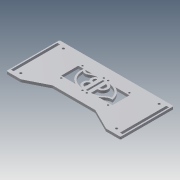
# Autodesk Inventor part: FrontPanel
Saved by Autodesk Inventor 2014 (Build 180170000, 170)
## iProperties
Created: 2015-01-19
Part Number: FrontPanel
Material: Generic
Document SubType Name: Modeling
Designer: Peele
Density: 1 g/cm^3
Appearance: White
Author: Peele
Autodesk Inventor part; units mm, degrees
ref_plane "YZ Plane" through (0, 0, 0) normal (1, 0, 0) x (0, 1, 0)
ref_plane "XZ Plane" through (0, 0, 0) normal (0, 1, 0) x (-1, 0, 0)
ref_plane "XY Plane" through (0, 0, 0) normal (0, 0, 1) x (1, 0, 0)
sketch "Sketch1" plane through (0, 0, 0) normal (0, 0, 1) x (1, 0, 0)
  line L0 (0, 0) -> (0, 125)
  line L1 (0, 125) -> (268, 125)
  line L2 (268, 125) -> (268, 0)
  line L3 (268, 0) -> (0, 0)
  point P0 (134, 125)
  dimension "d1" = 125
  dimension "d2" = 268
  constraints: 8 end point, 2 horizontal, 2 vertical, 1 midpoint
  measures "d1" distance of L1.end L2.end
  measures "d2" distance of L2.end L0.start
extrude "Extrusion1" add sketch "Sketch1" along normal blind 6
sketch "Sketch2" plane through (0, 0, 6) normal (0, 0, 1) x (1, 0, 0)
  line L0 (0, 0) -> (268, 0) projected
  line L1 (268, 0) -> (268, 125) projected
  line L2 (34, 0) -> (84, 25)
  line L3 (84, 25) -> (184, 25)
  line L4 (184, 25) -> (234, 0)
  line L5 (234, 0) -> (34, 0)
  line L6 (0, 125) -> (0, 0) projected
  dimension "d6" = 25
  dimension "d7" = 34
  dimension "d9" = 50
  dimension "d47" = 34
  constraints: 8 end point, 2 point on line, 1 collinear, 1 equal length, 1 parallel
  measures "d6" distance between parallel lines of L0 L3
  measures "d7" distance from line of L4.end L1
  measures "d9" horizontal distance of L2.end L2.start
  measures "d47" distance from line of L6 L2.start
extrude "Extrusion2" cut sketch "Sketch2" against normal through all
sketch "Sketch7" plane through (0, 0, 6) normal (0, 0, 1) x (1, 0, 0)
  line L0 (268, 0) -> (268, 125) projected
  line L1 (268, 125) -> (0, 125) projected
  line L2 (0, 125) -> (0, 0) projected
  line L3 (0, 0) -> (34, 0) projected
  circle A0 centre (246.5, 12.5) radius 2.7
  circle A1 centre (246.5, 112.5) radius 2.7
  circle A2 centre (21.5, 12.5) radius 2.7
  circle A3 centre (21.5, 112.5) radius 2.7
  line L4 (2.875, 8.1) -> (9.125, 8.1)
  line L5 (9.125, 8.1) -> (9.125, 117)
  line L6 (9.125, 117) -> (2.875, 117)
  line L7 (2.875, 117) -> (2.875, 8.1)
  line L8 (2.875, 8.1) -> (9.125, 117) construction
  line L9 (9.125, 8.1) -> (2.875, 117) construction
  line L10 (258.875, 8.1) -> (265.125, 8.1)
  line L11 (265.125, 8.1) -> (265.125, 117)
  line L12 (265.125, 117) -> (258.875, 117)
  line L13 (258.875, 117) -> (258.875, 8.1)
  line L14 (258.875, 8.1) -> (265.125, 117) construction
  line L15 (265.125, 8.1) -> (258.875, 117) construction
  point P0 (6, 62.55)
  point P1 (262, 62.55)
  point P2 (6, 62.55)
  point P3 (262, 62.55)
  dimension "d48" = 21.5
  dimension "d49" = 21.5
  dimension "d50" = 12.5
  dimension "d51" = 12.5
  dimension "d56" = 2.875
  dimension "d57" = 6.25
  dimension "d58" = 2.875
  dimension "d60" = 8
  dimension "d61" = 5.4
  dimension "d62" = 108.9
  dimension "d66" = 8.1
  constraints: 24 end point, 6 midpoint, 4 centre point, 4 parallel, 3 equal radius, 3 horizontal alignment, 2 equal length, 2 horizontal, 2 perpendicular, 2 vertical alignment
  measures "d48" distance from line of A3.centre L2
  measures "d49" distance from line of A1.centre L0
  measures "d50" distance from line of A3.centre L1
  measures "d51" distance from line of A2.centre L3
  measures "d56" distance between parallel lines of L2 L7
  measures "d57" distance of L5.end L6.end
  measures "d58" distance between parallel lines of L11 L0
  measures "d60" distance between parallel lines of L1 L6
  measures "d61" diameter of A3
  measures "d62" distance of L4.end L5.end
  measures "d66" distance between parallel lines of L4 L3
extrude "Extrusion5" cut sketch "Sketch7" against normal through all
fillet "Fillet1" radius 2 8 edges at (268, 125, 3) (268, 0, 3) (234, 0, 3) (184, 25, 3) (84, 25, 3) (34, 0, 3) (0, 0, 3) (0, 125, 3)
sketch "Sketch8" plane through (0, 0, 6) normal (0, 0, 1) x (1, 0, 0)
  line L0 (9.125, 8.1) -> (2.875, 8.1) projected
  line L1 (84.4721, 25) -> (183.5279, 25) projected
  line L2 (266, 125) -> (2, 125) projected
  line L3 (79, 50) -> (129, 50) construction
  line L4 (129, 50) -> (129, 100) construction
  line L5 (129, 100) -> (79, 100) construction
  line L6 (79, 100) -> (79, 50) construction
  line L7 (79, 50) -> (129, 100) construction
  line L8 (129, 50) -> (79, 100) construction
  line L9 (139, 50) -> (189, 50) construction
  line L10 (189, 50) -> (189, 100) construction
  line L11 (189, 100) -> (139, 100) construction
  line L12 (139, 100) -> (139, 50) construction
  line L13 (139, 50) -> (189, 100) construction
  line L14 (189, 50) -> (139, 100) construction
  line L15 (104, 75) -> (164, 75) construction
  line L16 (134, 75) -> (134, 25) construction
  circle A0 centre (79, 100) radius 2.15
  circle A1 centre (129, 100) radius 2.15
  circle A2 centre (139, 100) radius 2.15
  circle A3 centre (189, 100) radius 2.15
  circle A4 centre (189, 50) radius 2.15
  circle A5 centre (139, 50) radius 2.15
  circle A6 centre (129, 50) radius 2.15
  circle A7 centre (79, 50) radius 2.15
  point P0 (0, 0)
  dimension "d67" = 50
  dimension "d68" = 60
  dimension "d69" = 100
  dimension "d70" = 25
  dimension "d71" = 4.3
  constraints: 28 end point, 8 centre point, 8 coincident, 7 equal radius, 6 midpoint, 5 parallel, 3 equal length, 3 perpendicular, 2 horizontal, 1 vertical
  measures "d67" distance of L4.end L5.end
  measures "d68" distance of L15.end L15.start
  measures "d69" distance between parallel lines of L2 L1
  measures "d70" distance between parallel lines of L2 L5
  measures "d71" diameter of A3
extrude "Extrusion6" cut sketch "Sketch8" against normal blind 10
sketch "Sketch9" plane through (0, 0, 6) normal (0, 0, 1) x (1, 0, 0)
  circle A0 centre (79, 100) radius 2.15 projected
  circle A1 centre (79, 50) radius 2.15 projected
  line L0 (9.125, 117) -> (9.125, 8.1) projected
  line L1 (9.125, 8.1) -> (2.875, 8.1) projected
  line L2 (84.4721, 25) -> (183.5279, 25) projected
  line L3 (132, 55) -> (136, 55)
  line L4 (136, 55) -> (136, 95)
  line L5 (136, 95) -> (132, 95)
  line L6 (132, 95) -> (132, 55)
  line L7 (132, 55) -> (136, 95) construction
  line L8 (136, 55) -> (132, 95) construction
  line L9 (134, 25) -> (134, 75) construction
  line L10 (144, 90) -> (144, 75)
  arc A2 (144, 75) -> (144, 90) centre (144, 82.5) ccw
  arc A3 (144, 70) -> (144, 95) centre (144, 82.5) ccw
  line L11 (144, 70) -> (144, 55)
  arc A4 (178, 70) -> (144, 95) centre (144, 59.38) ccw
  arc A5 (178, 70) -> (166, 64) centre (181.2699, 48.4602) ccw
  arc A6 (144, 55) -> (166, 64) centre (144, 86.3889) ccw
  line L12 (144, 95) -> (136, 95) construction
  line L13 (136, 55) -> (144, 55) construction
  line L14 (161.3482, 95) -> (194, 95)
  line L15 (194, 95) -> (194, 55)
  line L16 (194, 55) -> (160.3435, 55)
  arc A7 (183.0358, 66.1589) -> (161.3482, 95) centre (144, 59.38) ccw
  arc A8 (160.3435, 55) -> (168.8035, 61.1469) centre (144, 86.3889) ccw
  arc A9 (183.0358, 66.1589) -> (168.8035, 61.1469) centre (181.2699, 48.4602) ccw
  line L17 (124, 75) -> (124, 60)
  line L18 (124, 90) -> (124, 80)
  arc A10 (124, 90) -> (124, 80) centre (124, 85) ccw
  arc A11 (124, 75) -> (124, 60) centre (124, 67.5) ccw
  arc A12 (117.0015, 77.8571) -> (124, 55) centre (124, 67.5) ccw
  arc A13 (124, 95) -> (117.0015, 77.8571) centre (124, 85) ccw
  line L19 (132, 95) -> (124, 95) construction
  line L20 (132, 55) -> (124, 55) construction
  arc A14 (124, 95) -> (104, 89) centre (124, 58.6667) ccw
  arc A15 (90, 90) -> (104, 89) centre (97.652, 98.6278) ccw
  arc A16 (90, 90) -> (124, 55) centre (124, 89.0143) ccw
  line L21 (86.4599, 95) -> (74, 95)
  line L22 (74, 95) -> (74, 55)
  line L23 (74, 55) -> (107.0261, 55)
  arc A17 (86.4599, 95) -> (107.0261, 55) centre (124, 89.0143) ccw
  arc A18 (91.051, 95) -> (101.7982, 92.3394) centre (97.652, 98.6278) ccw
  arc A19 (106.4881, 95) -> (101.7982, 92.3394) centre (124, 58.6667) ccw
  line L24 (91.051, 95) -> (106.4881, 95)
  point P0 (0, 0)
  point P1 (140, 55)
  dimension "d74" = 4
  dimension "d75" = 40
  dimension "d76" = 50
  dimension "d77" = 25
  dimension "d78" = 12.5
  dimension "d79" = 5
  dimension "d80" = 8
  dimension "d81" = 22
  dimension "d82" = 15
  dimension "d83" = 34
  dimension "d84" = 9
  dimension "d85" = 4
  dimension "d86" = 4
  dimension "d87" = 60
  dimension "d88" = 8
  dimension "d89" = 5
  dimension "d90" = 10
  dimension "d91" = 5
  dimension "d92" = 34
  dimension "d93" = 35
  dimension "d94" = 20
  dimension "d95" = 6
  dimension "d96" = 60
  dimension "d97" = 4
  dimension "d99" = 4
  constraints: 45 end point, 36 point on circle, 18 centre point, 12 parallel, 11 tangent, 9 collinear, 9 concentric, 5 horizontal, 4 midpoint, 4 perpendicular, 1 equal radius, 1 point on line, 1 vertical
  measures "d74" distance of L4.end L5.end
  measures "d75" distance of L5.end L3.start
  measures "d76" distance of A1.centre A0.centre
  measures "d77" vertical distance of L9.end A0.centre
  measures "d78" radius of A3
  measures "d79" radial gap between concentric circles of A3 A2
  measures "d80" distance between parallel lines of L4 L10
  measures "d81" distance from line of A5.end L11
  measures "d82" distance from line of A4.start L3
  measures "d83" distance from line of A4.start L11
  measures "d84" distance from line of A5.end L3
  measures "d85" radial gap between concentric circles of A7 A4
  measures "d86" radial gap between concentric circles of A6 A8
  measures "d87" distance from line of L9.end L15
  measures "d88" distance between parallel lines of L18 L6
  measures "d89" radial gap between concentric circles of A12 A11
  measures "d90" radius of A13
  measures "d91" radial gap between concentric circles of A13 A10
  measures "d92" distance from line of A15.start L17
  measures "d93" distance from line of A15.start L20
  measures "d94" distance from line of A14.end L18
  measures "d95" distance from line of A14.end L19
  measures "d96" distance from line of L22 L9.end
  measures "d97" radial gap between concentric circles of A16 A17
  measures "d99" radial gap between concentric circles of A18 A15
extrude "Extrusion7" cut sketch "Sketch9" against normal blind 10 contours L6 L5 L4 L3 | A2 L10 | A3 A4 A5 A6 L11 | L14 L15 L16 A8 A9 A7 | L17 A11 | L18 A10 | A12 A16 A15 A14 A13 | A17 L23 L22 L21 | L24 A19 A18
equation "\"d7\" = d47"
equation "\"d49\" = d48"
equation "\"d51\" = d50"
equation "\"d58\" = d56"
equation "\"d70\" = -0.5 * d67 + 0.5 * d69"
equation "\"d77\" = 0.5 * d76"
equation "\"d86\" = d85"
equation "\"d89\" = d79"
equation "\"d91\" = d79"
equation "\"d97\" = d85"
body "Solid1"
